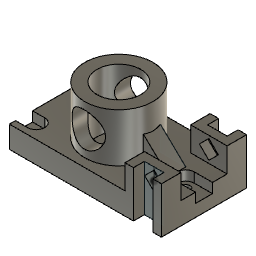
drawing_18 v1 (Autodesk Fusion 360 design; units mm, degrees)
Autodesk Fusion 360 part; units mm, degrees
sketch "Sketch1" plane through (0, 0, 0) normal (0, 0, 1) x (1, 0, 0)
  line L0 (0, 0) -> (62.5, 0) construction
  line L1 (0, 0) -> (-62.5, 0) construction
  line L2 (-62.5, 0) -> (-62.5, 35) construction
  line L3 (62.5, 0) -> (62.5, -35) construction
  line L4 (-62.5, 35) -> (62.5, 35)
  line L5 (62.5, 35) -> (62.5, -35)
  line L6 (62.5, -35) -> (-62.5, -35)
  line L7 (-62.5, -35) -> (-62.5, 35)
  dimension "d1" = 62.5
  dimension "d2" = 62.5
  dimension "d3" = 35
  dimension "d4" = 35
  constraint coincident L0.start L1.start
  constraint horizontal L0
  constraint parallel L0 L1
  constraint perpendicular L1 L2
  constraint perpendicular L0 L3
  constraint horizontal L4
  constraint vertical L5
  constraint horizontal L6
  constraint vertical L7
  measures "d1" distance of L0.start L0.end
  measures "d2" distance of L0.start L1.end
  measures "d3" distance of L1.end L2.end
  measures "d4" distance of L0.end L3.end
extrude "Extrude1" add sketch "Sketch1" along normal blind 18 makes body 1
sketch "Sketch2" plane through (0, 0, 18) normal (0, 0, 1) x (-1, 0, 0)
  line L0 (62.5, 35) -> (-62.5, 35)
  line L1 (-62.5, 35) -> (-62.5, -35)
  line L2 (-62.5, -35) -> (62.5, -35)
  line L3 (62.5, -35) -> (62.5, 35)
  line L4 (62.5, 0) -> (62.5, -23) construction
  line L5 (62.5, 0) -> (62.5, 23) construction
  line L6 (62.5, -23) -> (52.5, -23) construction
  line L7 (56.5, 23) -> (52.5, 23) construction
  circle A0 centre (52.5, -23) radius 4
  circle A1 centre (52.5, 23) radius 4
  circle A2 centre (52.5, -23) radius 7
  line L8 (52.4737, -30) -> (62.5, -30)
  line L9 (62.5, -30) -> (62.5, -16)
  line L10 (62.5, -16) -> (52.5, -16)
  line L11 (62.5, 23) -> (62.5, 16)
  line L12 (62.5, 23) -> (62.5, 30)
  line L13 (62.5, 30) -> (52.5, 30)
  line L14 (62.5, 16) -> (52.5, 16)
  arc A3 (52.5, 30) -> (52.5018, 16) centre (52.5, 23) ccw
  dimension "d9" = 10
  dimension "d10" = 10
  dimension "d11" = 8
  dimension "d12" = 8
  dimension "d13" = 14
  dimension "d14" = 14
  dimension "d15" = 14
  dimension "d16" = 7
  dimension "d17" = 7
  constraint midpoint L3 L4.start
  constraint parallel L3 L4
  constraint parallel L3 L5
  constraint perpendicular L4 L6
  constraint perpendicular L5 L7
  constraint coincident L6.end A0.centre
  constraint coincident L7.end A1.centre
  constraint concentric A0 A2
  constraint concentric A1 A3
  constraint coincident A2 L8.start
  constraint coincident L3 L8.end
  constraint perpendicular L3 L8
  constraint perpendicular L8 L9
  constraint coincident A2 L10.end
  constraint tangent A2 L10
  constraint perpendicular L7 L11
  constraint tangent L13 A3
  constraint coincident L14.end A3
  constraint coincident A1 L7.start
  constraint coincident L14 A3.end
  measures "d9" distance of L4.end L6.end
  measures "d10" distance of L5.end L7.end
  measures "d11" diameter of A0
  measures "d12" diameter of A1
  measures "d13" diameter of A2
  measures "d14" diameter of A3
  measures "d15" distance of L8.end L9.end
  measures "d16" distance of L5.end L11.end
  measures "d17" distance of L5.end L12.end
extrude "Extrude2" cut sketch "Sketch2" against normal blind 8 contours L3 L11 L12 L13 L14 A3 | A1 bodies 1
extrude "Extrude3" cut 1 faces at (-20.8333, 35, 6) along direction (0, -1, 0) blind 35 on bodies 1 bodies 1
mirror "Mirror1" about plane through (-62.5, 0, 0) normal (0, 1, 0) of bodies 1 merged
sketch "Sketch3" plane through (0, 0, 18) normal (0, 0, 1) x (-1, 0, 0)
  line L0 (62.5, -16) -> (62.5, 16)
  line L1 (62.5, 16) -> (52.5018, 16)
  arc A0 (52.5, 30) -> (52.5018, 16) centre (52.5, 23) ccw
  line L2 (52.5, 30) -> (62.5, 30)
  line L3 (62.5, 30) -> (62.5, 35)
  line L4 (62.5, 35) -> (-62.5, 35)
  line L5 (-62.5, 35) -> (-62.5, -35)
  line L6 (-62.5, -35) -> (62.5, -35)
  line L7 (62.5, -35) -> (62.5, -30)
  line L8 (62.5, -30) -> (52.5, -30)
  arc A1 (52.5018, -16) -> (52.5, -30) centre (52.5, -23) ccw
  line L9 (52.5018, -16) -> (62.5, -16)
  line L10 (62.5, -30) -> (62.5, -16)
  line L11 (62.5, -16) -> (52.5018, -16)
  arc A2 (52.5018, -16) -> (52.5, -30) centre (52.5, -23) ccw
  line L12 (52.5, -30) -> (62.5, -30)
  line L13 (62.5, 16) -> (62.5, 30)
  line L14 (62.5, 30) -> (52.5, 30)
  arc A3 (52.5, 30) -> (52.5018, 16) centre (52.5, 23) ccw
  line L15 (52.5018, 16) -> (62.5, 16)
  circle A4 centre (52.5, -23) radius 4
  circle A5 centre (52.5, 23) radius 4
  dimension "d24" = 8
  dimension "d25" = 8
  constraint concentric A2 A4
  constraint concentric A3 A5
  measures "d24" diameter of A4
  measures "d25" diameter of A5
  measures "d72" diameter of origin
  measures "d75" diameter of origin
  measures "d78" diameter of origin
extrude "Extrude4" cut sketch "Sketch3" against normal blind 134 contours A4 | A5 bodies 1
sketch "Sketch4" plane through (0, 0, 18) normal (0, 0, 1) x (-1, 0, 0)
  line L0 (62.5, -16) -> (62.5, 16)
  line L1 (62.5, 16) -> (52.5018, 16)
  arc A0 (52.5, 30) -> (52.5018, 16) centre (52.5, 23) ccw
  line L2 (52.5, 30) -> (62.5, 30)
  line L3 (62.5, 30) -> (62.5, 35)
  line L4 (62.5, 35) -> (-62.5, 35)
  line L5 (-62.5, 35) -> (-62.5, -35)
  line L6 (-62.5, -35) -> (62.5, -35)
  line L7 (62.5, -35) -> (62.5, -30)
  line L8 (62.5, -30) -> (52.5, -30)
  arc A1 (52.5018, -16) -> (52.5, -30) centre (52.5, -23) ccw
  line L9 (52.5018, -16) -> (62.5, -16)
  line L10 (-62.5, -35) -> (-47.5, -35) construction
  line L11 (-62.5, 35) -> (-47.5, 35) construction
  line L12 (-62.5, 0) -> (-62.5, -26) construction
  line L13 (-62.5, 0) -> (-62.5, 26) construction
  line L14 (-47.5, -35) -> (-39.5, -35) construction
  line L15 (-47.5, -35) -> (-55.5, -35) construction
  line L16 (-47.5, 35) -> (-55.5, 35) construction
  line L17 (-47.5, 35) -> (-39.5, 35) construction
  line L18 (-39.5, 35) -> (-55.5, 35) construction
  line L19 (-55.5, 35) -> (-55.5, 26) construction
  line L20 (-55.5, 26) -> (-39.5, 26) construction
  line L21 (-39.5, 26) -> (-39.5, 35) construction
  line L22 (-39.5, 35) -> (-55.5, 35)
  line L23 (-55.5, 35) -> (-55.5, 26)
  line L24 (-55.5, 26) -> (-39.5, 26)
  line L25 (-39.5, 26) -> (-39.5, 35)
  line L26 (-55.5, -35) -> (-39.5, -35)
  line L27 (-39.5, -35) -> (-39.5, -26)
  line L28 (-39.5, -26) -> (-55.5, -26)
  line L29 (-55.5, -26) -> (-55.5, -35)
  dimension "d28" = 15
  dimension "d29" = 15
  dimension "d30" = 26
  dimension "d31" = 26
  dimension "d32" = 8
  dimension "d33" = 8
  dimension "d34" = 8
  dimension "d35" = 8
  dimension "d36" = 16
  constraint coincident L5.end L6.start
  constraint perpendicular L5 L10
  constraint coincident L4.end L5.start
  constraint perpendicular L5 L11
  constraint midpoint L5 L12.start
  constraint parallel L5 L12
  constraint parallel L5 L13
  constraint parallel L6 L14
  constraint parallel L6 L15
  constraint parallel L4 L16
  constraint parallel L16 L17
  constraint horizontal L18
  constraint vertical L19
  constraint horizontal L20
  constraint vertical L21
  constraint horizontal L22
  constraint vertical L23
  constraint horizontal L24
  constraint vertical L25
  constraint horizontal L26
  constraint vertical L27
  constraint horizontal L28
  constraint vertical L29
  measures "d28" distance of L5.end L10.end
  measures "d29" distance of L4.end L11.end
  measures "d30" distance of L12.start L12.end
  measures "d31" distance of L12.start L13.end
  measures "d32" distance of L10.end L14.end
  measures "d33" distance of L10.end L15.end
  measures "d34" distance of L11.end L16.end
  measures "d35" distance of L11.end L17.end
  measures "d36" distance of L17.end L16.end
extrude "Extrude5" cut sketch "Sketch4" against normal blind 51 contours L6 L26 L27 L28 L29 | L4 L22 L23 L24 L25 bodies 1
sketch "Sketch5" plane through (0, 0, 18) normal (0, 0, 1) x (-1, 0, 0)
  line L0 (-39.5, -26) -> (-39.5, -35)
  line L1 (-39.5, -35) -> (62.5, -35)
  line L2 (62.5, -35) -> (62.5, -30)
  line L3 (62.5, -30) -> (52.5, -30)
  arc A0 (52.5018, -16) -> (52.5, -30) centre (52.5, -23) ccw
  line L4 (52.5018, -16) -> (62.5, -16)
  line L5 (62.5, -16) -> (62.5, 16)
  line L6 (62.5, 16) -> (52.5018, 16)
  arc A1 (52.5, 30) -> (52.5018, 16) centre (52.5, 23) ccw
  line L7 (52.5, 30) -> (62.5, 30)
  line L8 (62.5, 30) -> (62.5, 35)
  line L9 (62.5, 35) -> (-39.5, 35)
  line L10 (-39.5, 35) -> (-39.5, 26)
  line L11 (-39.5, 26) -> (-55.5, 26)
  line L12 (-55.5, 26) -> (-55.5, 35)
  line L13 (-55.5, 35) -> (-62.5, 35)
  line L14 (-62.5, 35) -> (-62.5, -35)
  line L15 (-62.5, -35) -> (-55.5, -35)
  line L16 (-55.5, -35) -> (-55.5, -26)
  line L17 (-55.5, -26) -> (-39.5, -26)
  line L18 (-62.5, 0) -> (-62.5, -19) construction
  line L19 (-62.5, 0) -> (-62.5, 19) construction
  line L20 (-39.5, 35) -> (-32.5, 35) construction
  line L21 (-32.5, -35) -> (-39.5, -35) construction
  line L22 (-62.5, -19) -> (-32.5, -19)
  line L23 (-32.5, -19) -> (-32.5, -35)
  line L24 (-32.5, 19) -> (-62.5, 19)
  line L25 (-32.5, 35) -> (-32.5, 19)
  dimension "d39" = 19
  dimension "d40" = 19
  dimension "d41" = 7
  constraint midpoint L14 L18.start
  constraint parallel L14 L18
  constraint parallel L14 L19
  constraint coincident L9.end L10.start
  constraint perpendicular L10 L20
  constraint coincident L1 L21.start
  constraint coincident L0.end L1.start
  constraint perpendicular L0 L21
  constraint perpendicular L14 L22
  constraint perpendicular L1 L23
  constraint perpendicular L19 L24
  constraint perpendicular L20 L25
  measures "d39" distance of L18.start L18.end
  measures "d40" distance of L18.start L19.end
  measures "d41" distance of L9.end L20.end
extrude "Extrude6" cut sketch "Sketch5" against normal blind 8 contours L0 L1 L14 L15 L16 L17 L22 L23 | L9 L10 L11 L12 L13 L14 L24 L25 bodies 1
sketch "Sketch6" plane through (0, 0, 18) normal (0, 0, 1) x (-1, 0, 0)
  line L0 (-32.5, 19) -> (-62.5, 19)
  line L1 (-62.5, 19) -> (-62.5, -19)
  line L2 (-62.5, -19) -> (-32.5, -19)
  line L3 (-32.5, -19) -> (-32.5, -35)
  line L4 (-32.5, -35) -> (62.5, -35)
  line L5 (62.5, -35) -> (62.5, -30)
  line L6 (62.5, -30) -> (52.5, -30)
  arc A0 (52.5018, -16) -> (52.5, -30) centre (52.5, -23) ccw
  line L7 (52.5018, -16) -> (62.5, -16)
  line L8 (62.5, -16) -> (62.5, 16)
  line L9 (62.5, 16) -> (52.5018, 16)
  arc A1 (52.5, 30) -> (52.5018, 16) centre (52.5, 23) ccw
  line L10 (52.5, 30) -> (62.5, 30)
  line L11 (62.5, 30) -> (62.5, 35)
  line L12 (62.5, 35) -> (-32.5, 35)
  line L13 (-32.5, 35) -> (-32.5, 19)
  line L14 (-62.5, 0) -> (-62.5, -7) construction
  line L15 (-62.5, 0) -> (-62.5, 7) construction
  line L16 (-62.5, -7) -> (-47.5, -7)
  line L17 (-62.5, 7) -> (-47.5, 7)
  line L18 (-62.5, 0) -> (-47.5, 0) construction
  arc A2 (-47.5, -7) -> (-47.5, 7) centre (-47.5, 0) ccw
  dimension "d44" = 7
  dimension "d45" = 7
  dimension "d48" = 15
  constraint midpoint L1 L14.start
  constraint parallel L1 L14
  constraint parallel L1 L15
  constraint perpendicular L1 L16
  constraint perpendicular L1 L17
  constraint perpendicular L1 L18
  constraint coincident L18.end A2.centre
  constraint tangent L16 A2
  measures "d44" distance of L14.start L14.end
  measures "d45" distance of L14.start L15.end
  measures "d48" distance of L14.start L18.end
extrude "Extrude7" cut sketch "Sketch6" against normal blind 8 contours L1 L16 L17 A2 bodies 1
extrude "Extrude8" add 2 faces at (44.8333, -21.3333, 10) (44.8333, 21.3333, 10) along direction (0, 0, 1) blind 28 on bodies 1 bodies 1
sketch "Sketch10" plane through (0, -26, 0) normal (0, -1, 0) x (1, 0, 0)
  line L0 (39.5, 38) -> (39.5, 0)
  line L1 (39.5, 0) -> (55.5, 0)
  line L2 (55.5, 0) -> (55.5, 38)
  line L3 (55.5, 38) -> (39.5, 38)
  line L4 (47.5, 38) -> (47.5, 28) construction
  dimension "d63" = 10
  constraint midpoint L3 L4.start
  constraint perpendicular L3 L4
  measures "d63" distance of L4.start L4.end
sketch "Sketch11" plane through (0, 0, 0) normal (0, 1, 0) x (1, 0, 0)
  line L0 (80, -35) -> (91, -35)
  line L1 (91, -35) -> (91, -24)
  line L2 (91, -24) -> (80, -24)
  line L3 (80, -24) -> (80, -35)
  dimension "d64" = 11
  dimension "d65" = 11
  constraint horizontal L0
  constraint vertical L1
  constraint horizontal L2
  constraint vertical L3
  measures "d64" distance of L0.start L0.end
  measures "d65" distance of L0.start L2.end
extrude "Extrude11" add sketch "Sketch11" along normal mid plane 140 separate body makes body 2
move_body "Move1" bodies 2 to x (0.707107, 0, 0.707107) y (0, 1, 0) z (-0.707107, 0, 0.707107) at (45.902, 0, -51.8173)
move_body "Align1" bodies 2 to x (1, 0, 0) y (0, 1, 0) z (0, 0, 1) at (-38, 44, -1.5)
move_body "Move2" bodies 2 to x (1, 0, 0) y (0, 1, 0) z (0, 0, 1) at (0, -35, 0)
combine "Combine1" operation cut target body 1 tool bodies 2
sketch "Sketch12" plane through (0, 0, 10) normal (0, 0, 1) x (-1, 0, 0)
  line L0 (-62.5, 7) -> (-62.5, -7)
  line L1 (-62.5, -7) -> (-47.5, -7)
  arc A0 (-47.5, -7) -> (-47.5, 7) centre (-47.5, 0) ccw
  line L2 (-47.5, 7) -> (-62.5, 7)
  circle A1 centre (-47.5, 0) radius 3.5
  dimension "d68" = 7
  constraint concentric A0 A1
  measures "d68" diameter of A1
extrude "Extrude12" cut sketch "Sketch12" against normal blind 18 contours A1 bodies 1
sketch "Sketch13" plane through (0, 0, 18) normal (0, 0, 1) x (-1, 0, 0)
  line L0 (-62.5, 7) -> (-47.5, 7)
  arc A0 (-47.5, -7) -> (-47.5, 7) centre (-47.5, 0) ccw
  line L1 (-47.5, -7) -> (-62.5, -7)
  line L2 (-62.5, -7) -> (-62.5, -19)
  line L3 (-62.5, -19) -> (-32.5, -19)
  line L4 (-32.5, -19) -> (-32.5, -35)
  line L5 (-32.5, -35) -> (62.5, -35)
  line L6 (62.5, -35) -> (62.5, -30)
  line L7 (62.5, -30) -> (52.5, -30)
  arc A1 (52.5018, -16) -> (52.5, -30) centre (52.5, -23) ccw
  line L8 (52.5018, -16) -> (62.5, -16)
  line L9 (62.5, -16) -> (62.5, 16)
  line L10 (62.5, 16) -> (52.5018, 16)
  arc A2 (52.5, 30) -> (52.5018, 16) centre (52.5, 23) ccw
  line L11 (52.5, 30) -> (62.5, 30)
  line L12 (62.5, 30) -> (62.5, 35)
  line L13 (62.5, 35) -> (-32.5, 35)
  line L14 (-32.5, 35) -> (-32.5, 19)
  line L15 (-32.5, 19) -> (-62.5, 19)
  line L16 (-62.5, 19) -> (-62.5, 7)
  line L17 (-39.5, 35) -> (-39.5, 26)
  line L18 (-39.5, 26) -> (-55.5, 26)
  line L19 (-55.5, 26) -> (-55.5, 35)
  line L20 (-55.5, 35) -> (-62.5, 35)
  line L21 (-62.5, 35) -> (-62.5, 19)
  line L22 (-62.5, 19) -> (-32.5, 19)
  line L23 (-32.5, 19) -> (-32.5, 35)
  line L24 (-32.5, 35) -> (-39.5, 35)
  line L25 (-62.5, 35) -> (7.5, 35) construction
  circle A3 centre (7.5, 0) radius 28
  point P0 (7.5, 0)
  dimension "d71" = 70
  dimension "d72" = 56
  constraint coincident L20.end L21.start
  constraint perpendicular L19 L25
  constraint coincident P0 A3.centre
  measures "d71" distance of L20.end L25.end
  measures "d72" diameter of A3
extrude "Extrude13" add sketch "Sketch13" along normal blind 40 contours A3 bodies 1
sketch "Sketch14" plane through (0, 0, 58) normal (0, 0, 1) x (-1, 0, 0)
  circle A0 centre (7.5, 0) radius 28
  circle A1 centre (7.5, 0) radius 18
  dimension "d75" = 36
  constraint concentric A0 A1
  measures "d75" diameter of A1
extrude "Extrude14" cut sketch "Sketch14" against normal blind 48 contours A1 bodies 1
sketch "Sketch15" plane through (0, 0, 10) normal (0, 0, 1) x (-1, 0, 0)
  circle A0 centre (7.5, 0) radius 18
  circle A1 centre (7.5, 0) radius 9
  dimension "d78" = 18
  constraint concentric A0 A1
  measures "d78" diameter of A1
extrude "Extrude15" cut sketch "Sketch15" against normal blind 50 contours A1 bodies 1
sketch "Sketch16" plane through (0, 0, 18) normal (0, 0, 1) x (-1, 0, 0)
  circle A0 centre (7.5, 0) radius 28
  line L0 (-62.5, 7) -> (-47.5, 7)
  arc A1 (-47.5, -7) -> (-47.5, 7) centre (-47.5, 0) ccw
  line L1 (-47.5, -7) -> (-62.5, -7)
  line L2 (-62.5, -7) -> (-62.5, -19)
  line L3 (-62.5, -19) -> (-32.5, -19)
  line L4 (-32.5, -19) -> (-32.5, -35)
  line L5 (-32.5, -35) -> (62.5, -35)
  line L6 (62.5, -35) -> (62.5, -30)
  line L7 (62.5, -30) -> (52.5, -30)
  arc A2 (52.5018, -16) -> (52.5, -30) centre (52.5, -23) ccw
  line L8 (52.5018, -16) -> (62.5, -16)
  line L9 (62.5, -16) -> (62.5, 16)
  line L10 (62.5, 16) -> (52.5018, 16)
  arc A3 (52.5, 30) -> (52.5018, 16) centre (52.5, 23) ccw
  line L11 (52.5, 30) -> (62.5, 30)
  line L12 (62.5, 30) -> (62.5, 35)
  line L13 (62.5, 35) -> (-32.5, 35)
  line L14 (-32.5, 35) -> (-32.5, 19)
  line L15 (-32.5, 19) -> (-62.5, 19)
  line L16 (-62.5, 19) -> (-62.5, 7)
  circle A4 centre (-47.5, 0) radius 3.5 construction
  line L17 (-62.5, 7) -> (-62.5, -7) construction
  line L18 (-62.5, -7) -> (-47.5, -7) construction
  arc A5 (-47.5, -7) -> (-47.5, 7) centre (-47.5, 0) ccw construction
  line L19 (-47.5, 7) -> (-62.5, 7) construction
  line L20 (-62.5, 0) -> (-40.5, 0) construction
  line L21 (-40.5, 0) -> (-40.5, -7)
  line L22 (-40.5, -7) -> (-40.5, 7)
  line L23 (-40.5, 7) -> (-13.5, 7)
  line L24 (-13.5, 7) -> (-13.5, -7)
  line L25 (-13.5, -7) -> (-40.5, -7)
  line L26 (-40.5, -7) -> (-40.5, 7)
  dimension "d81" = 7
  dimension "d82" = 14
  dimension "d83" = 27
  dimension "d84" = 14
  constraint midpoint L17 L20.start
  constraint midpoint A1 L20.end
  constraint perpendicular L20 L21
  constraint perpendicular L20 L22
  constraint horizontal L23
  constraint vertical L24
  constraint horizontal L25
  constraint vertical L26
  measures "d81" distance of L20.end L21.end
  measures "d82" distance of L21.end L22.end
  measures "d83" distance of L22.end L23.end
  measures "d84" distance of L22.end L21.end
extrude "Extrude16" add sketch "Sketch16" along normal blind 20 separate body contours A0 L23 L24 L25 | A0 L21 L22 L23 L25 L26 picked at (-15.8333, 0) makes body 3
sketch "Sketch17" plane through (0, 0, 38) normal (0, 0, 1) x (-1, 0, 0)
  line L0 (-40.5, -7) -> (-13.5, -7)
  line L1 (-13.5, -7) -> (-13.5, 7)
  line L2 (-13.5, 7) -> (-40.5, 7)
  line L3 (-40.5, 7) -> (-40.5, -7)
  circle A0 centre (7.5, 0) radius 18
  circle A1 centre (7.5, 0) radius 28
extrude "Extrude17" add sketch "Sketch17" against normal blind 25 contours L0 L2 L3 A1 bodies 1 3
sketch "Sketch18" plane through (0, -7, 0) normal (0, -1, 0) x (1, 0, 0)
  line L0 (19.6109, 38) -> (19.6109, 18)
  line L1 (19.6109, 18) -> (40.5, 18)
  line L2 (40.5, 18) -> (40.5, 38)
  line L3 (40.5, 38) -> (19.6109, 38)
  line L4 (19.6109, 38) -> (40.5, 18)
  constraint coincident L0.start L3.end
  constraint coincident L1.end L2.start
extrude "Extrude18" cut sketch "Sketch18" against normal blind 20 contours L2 L3 L4 bodies 1
sketch "Sketch19" plane through (0, 7, 0) normal (0, 1, 0) x (-1, 0, 0)
  line L0 (-19.6109, 38) -> (-40.5, 18)
  line L1 (-40.5, 18) -> (-19.6109, 18)
  line L2 (-19.6109, 18) -> (-19.6109, 38)
extrude "Extrude19" add 1 faces at (-32.0624, 1.3911, 58) along direction (0, 0, -1) blind 36 on bodies 1 bodies 1
sketch "Sketch20" plane through (0, 35, 0) normal (0, 1, 0) x (-1, 0, 0)
  line L0 (-39.5, 38) -> (-39.5, 0)
  line L1 (-39.5, 0) -> (62.5, 0)
  line L2 (62.5, 0) -> (62.5, 18)
  line L3 (62.5, 18) -> (-32.5, 18)
  line L4 (-32.5, 18) -> (-32.5, 38)
  line L5 (-32.5, 38) -> (-39.5, 38)
  line L6 (35.5, 58) -> (-20.5, 58)
  line L7 (-19.6109, 38) -> (-19.6109, 18)
  line L8 (-19.6109, 18) -> (35.5, 18)
  line L9 (-19.6109, 18) -> (-19.6109, 38)
  line L10 (-20.5, 37.1487) -> (-19.6109, 38)
  line L11 (7.9446, 18) -> (7.9446, 38)
  circle A0 centre (7.9446, 38) radius 14
  dimension "d93" = 20
  dimension "d94" = 28
  constraint midpoint L8 L11.start
  constraint perpendicular L3 L11
  constraint coincident L11.end A0.centre
  measures "d93" distance of L11.start L11.end
  measures "d94" diameter of A0
extrude "Extrude20" cut sketch "Sketch20" against normal blind 88 contours A0 bodies 1
equation "d1 = ( 125 / 2 ) * 1 mm"
equation "d2 = ( 125 / 2 ) * 1 mm"
equation "d30 = ( 52 / 2 ) * 1 mm"
equation "d31 = ( 52 / 2 ) * 1 mm"
equation "d39 = ( 38 / 2 ) * 1 mm"
equation "d73 = 58 mm - 18 mm"
equation "d76 = -58 mm + 10 mm"
